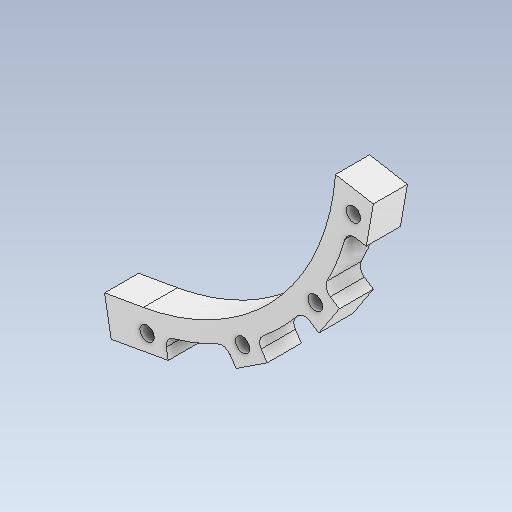
# Autodesk Inventor part: shell_5
Saved by Autodesk Inventor 2020 (Build 240168000, 168)
## iProperties
Created: 2020-07-15
Part Number: shell_5
Material: ABS Plastic
Document SubType Name: Modeling
Designer: psrobotics
Density: 1.06 g/cm^3
Appearance: Smooth - White
Author: psrobotics
Autodesk Inventor part; units mm, degrees
ref_plane "YZ Plane" through (0, 0, 0) normal (1, 0, 0) x (0, 1, 0)
ref_plane "XZ Plane" through (0, 0, 0) normal (0, 1, 0) x (-1, 0, 0)
ref_plane "XY Plane" through (0, 0, 0) normal (0, 0, 1) x (1, 0, 0)
sketch "Sketch1" plane through (0, 0, 0) normal (0, 0, 1) x (1, 0, 0)
  circle A0 centre (-48.56, 6.9152) radius 2.1 projected
  circle A1 centre (-32.9741, 22.501) radius 2.1 projected
  circle A2 centre (-69.0444, -1.2227) radius 2.1 projected
  circle A3 centre (-24.8362, 42.9855) radius 2.1 projected
  circle A4 centre (-46.3856, -8.3913) radius 8 projected
  line L0 (-28.6687, 48.4472) -> (-17.4995, 54.7179) projected
  arc A5 (-69.8258, 3.2089) -> (-28.6687, 48.4472) centre (-78.5082, 52.4493) ccw projected
  line L1 (-69.8258, 3.2089) -> (-78.128, 1.745) projected
  line L2 (-78.128, 1.745) -> (-74.0482, -21.3924) projected
  line L3 (-74.0482, -21.3924) -> (-70.3922, -20.7477) projected
  arc A6 (-70.3922, -20.7477) -> (-49.7861, -35.1763) centre (-46.3856, -8.3913) ccw projected
  line L4 (-49.7861, -35.1763) -> (-49.1414, -38.8323) projected
  line L5 (-49.1414, -38.8323) -> (-41.263, -37.4431) projected
  line L6 (-41.263, -37.4431) -> (4.3164, -53.3072) projected
  line L7 (4.3164, -53.3072) -> (1.8974, -59.9532) projected
  line L8 (1.8974, -59.9532) -> (17.5702, -63.2237) projected
  arc A7 (17.5702, -63.2237) -> (22.7521, -63.408) centre (22.2724, -3.9734) ccw projected
  line L9 (22.7521, -63.408) -> (22.7442, -62.4373) projected
  arc A8 (24.6597, -60.4229) -> (22.7442, -62.4373) centre (24.7442, -62.4211) ccw projected
  arc A9 (24.6597, -60.4229) -> (33.3265, -59.3815) centre (22.2724, -3.9734) ccw projected
  arc A10 (35.6646, -60.8847) -> (33.3265, -59.3815) centre (33.7178, -61.3428) ccw projected
  line L10 (35.6646, -60.8847) -> (35.9706, -62.1851) projected
  arc A11 (35.9706, -62.1851) -> (41.9803, -60.4344) centre (22.2724, -3.9734) ccw projected
  line L11 (41.9803, -60.4344) -> (52.856, -55.363) projected
  arc A12 (52.856, -55.363) -> (58.0602, -51.8846) centre (22.2724, -3.9734) ccw projected
  line L12 (58.0602, -51.8846) -> (57.2607, -50.8143) projected
  arc A13 (57.6121, -48.0569) -> (57.2607, -50.8143) centre (58.863, -49.6174) ccw projected
  arc A14 (57.6121, -48.0569) -> (63.9808, -42.0872) centre (22.2724, -3.9734) ccw projected
  arc A15 (66.7551, -41.9147) -> (63.9808, -42.0872) centre (65.4572, -43.4363) ccw projected
  line L13 (66.7551, -41.9147) -> (67.4937, -42.5447) projected
  arc A16 (67.4937, -42.5447) -> (70.6833, -38.4566) centre (22.2724, -3.9734) ccw projected
  line L14 (70.6833, -38.4566) -> (78.2523, -24.3484) projected
  line L15 (78.2523, -24.3484) -> (71.6063, -21.9294) projected
  arc A17 (71.6063, -21.9294) -> (67.7387, 22.2766) centre (22.2724, -3.9734) ccw projected
  line L16 (67.7387, 22.2766) -> (73.8637, 25.8129) projected
  line L17 (73.8637, 25.8129) -> (63.9599, 38.3925) projected
  arc A18 (63.9599, 38.3925) -> (60.1088, 41.8646) centre (22.2724, -3.9734) ccw projected
  line L18 (60.1088, 41.8646) -> (59.4908, 41.1159) projected
  arc A19 (56.7287, 40.804) -> (59.4908, 41.1159) centre (57.9484, 42.389) ccw projected
  arc A20 (56.7287, 40.804) -> (49.4201, 45.5771) centre (22.2724, -3.9734) ccw projected
  arc A21 (48.5953, 48.2316) -> (49.4201, 45.5771) centre (50.3811, 47.3311) ccw projected
  line L19 (48.5953, 48.2316) -> (49.1968, 49.4245) projected
  arc A22 (49.1968, 49.4245) -> (43.4677, 51.9463) centre (22.2724, -3.9734) ccw projected
  line L20 (43.4677, 51.9463) -> (31.8766, 55.0521) projected
  arc A23 (31.8766, 55.0521) -> (25.6541, 55.7327) centre (22.2724, -3.9734) ccw projected
  line L21 (25.6541, 55.7327) -> (25.5786, 54.3989) projected
  arc A24 (23.537, 52.5125) -> (25.5786, 54.3989) centre (23.5818, 54.512) ccw projected
  arc A25 (23.537, 52.5125) -> (14.821, 52.0331) centre (22.2724, -3.9734) ccw projected
  arc A26 (12.5849, 53.6843) -> (14.821, 52.0331) centre (14.5573, 54.0157) ccw projected
  line L22 (12.5849, 53.6843) -> (12.4241, 54.6417) projected
  arc A27 (12.4241, 54.6417) -> (7.3529, 53.5603) centre (22.2724, -3.9734) ccw projected
  line L23 (7.3529, 53.5603) -> (-7.5139, 47.618) projected
  line L24 (-7.5139, 47.618) -> (-17.4995, 54.7179) projected
  circle A28 centre (-71.296, -16.8454) radius 1.5 projected
  circle A29 centre (18.8152, -59.8032) radius 1.5 projected
  circle A30 centre (53.4562, -50.8504) radius 1.5 projected
  circle A31 centre (60.8075, 36.5725) radius 1.5 projected
  circle A32 centre (28.5162, 51.9811) radius 1.5 projected
  circle A33 centre (9.173, 50.4079) radius 1.5 projected
  circle A34 centre (44.8423, 47.6065) radius 1.5 projected
  circle A35 centre (67.2628, -37.2117) radius 1.5 projected
  circle A36 centre (38.1378, -57.9935) radius 1.5 projected
  circle A37 centre (-45.81, -34.6909) radius 1.5 projected
  circle A38 centre (22.2724, -3.9734) radius 32.5 projected
  circle A39 centre (-78.5082, 52.4493) radius 5.9 projected
  circle A40 centre (-78.5082, 52.4493) radius 50
  circle A41 centre (-78.5082, 52.4493) radius 54
  line L25 (-78.5082, 52.4493) -> (-69.0444, -1.2227)
  line L26 (-78.5082, 52.4493) -> (-24.8362, 42.9855)
  point P0 (0, 0)
  point P1 (-25.3286, 43.0723)
  point P2 (-29.2678, 43.7669)
  point P3 (-69.1312, -0.7303)
  dimension "d0" = 100
  dimension "d1" = 108
  constraints: 4 end point, 2 centre point, 2 coincident
  measures "d0" diameter of A40
  measures "d1" diameter of A41
extrude "Extrusion1" add sketch "Sketch1" along normal blind 7.3 contours A41 A0 | A0 A41 A2 L25 A5 L26 A3 A1 | A1 A41 | A41 L25 A2 | A3 L26 A41 picked at (-49.1962, 7.731) picked at (-33.8814, 22.9981) picked at (-68.8495, -0.1546) picked at (-25.9043, 42.7906)
sketch "Sketch2" plane through (0, 0, 7.3) normal (0, 0, 1) x (1, 0, 0)
  circle A0 centre (-48.56, 6.9152) radius 2.1 projected
  circle A1 centre (-32.9741, 22.501) radius 2.1 projected
  circle A2 centre (-69.0444, -1.2227) radius 2.1 projected
  circle A3 centre (-24.8362, 42.9855) radius 2.1 projected
  circle A4 centre (-46.3856, -8.3913) radius 8 projected
  line L0 (-28.6687, 48.4472) -> (-17.4995, 54.7179) projected
  arc A5 (-69.8258, 3.2089) -> (-28.6687, 48.4472) centre (-78.5082, 52.4493) ccw projected
  line L1 (-69.8258, 3.2089) -> (-78.128, 1.745) projected
  line L2 (-78.128, 1.745) -> (-74.0482, -21.3924) projected
  line L3 (-74.0482, -21.3924) -> (-70.3922, -20.7477) projected
  arc A6 (-70.3922, -20.7477) -> (-49.7861, -35.1763) centre (-46.3856, -8.3913) ccw projected
  line L4 (-49.7861, -35.1763) -> (-49.1414, -38.8323) projected
  line L5 (-49.1414, -38.8323) -> (-41.263, -37.4431) projected
  line L6 (-41.263, -37.4431) -> (4.3164, -53.3072) projected
  line L7 (4.3164, -53.3072) -> (1.8974, -59.9532) projected
  line L8 (1.8974, -59.9532) -> (17.5702, -63.2237) projected
  arc A7 (17.5702, -63.2237) -> (22.7521, -63.408) centre (22.2724, -3.9734) ccw projected
  line L9 (22.7521, -63.408) -> (22.7442, -62.4373) projected
  arc A8 (24.6597, -60.4229) -> (22.7442, -62.4373) centre (24.7442, -62.4211) ccw projected
  arc A9 (24.6597, -60.4229) -> (33.3265, -59.3815) centre (22.2724, -3.9734) ccw projected
  arc A10 (35.6646, -60.8847) -> (33.3265, -59.3815) centre (33.7178, -61.3428) ccw projected
  line L10 (35.6646, -60.8847) -> (35.9706, -62.1851) projected
  arc A11 (35.9706, -62.1851) -> (41.9803, -60.4344) centre (22.2724, -3.9734) ccw projected
  line L11 (41.9803, -60.4344) -> (52.856, -55.363) projected
  arc A12 (52.856, -55.363) -> (58.0602, -51.8846) centre (22.2724, -3.9734) ccw projected
  line L12 (58.0602, -51.8846) -> (57.2607, -50.8143) projected
  arc A13 (57.6121, -48.0569) -> (57.2607, -50.8143) centre (58.863, -49.6174) ccw projected
  arc A14 (57.6121, -48.0569) -> (63.9808, -42.0872) centre (22.2724, -3.9734) ccw projected
  arc A15 (66.7551, -41.9147) -> (63.9808, -42.0872) centre (65.4572, -43.4363) ccw projected
  line L13 (66.7551, -41.9147) -> (67.4937, -42.5447) projected
  arc A16 (67.4937, -42.5447) -> (70.6833, -38.4566) centre (22.2724, -3.9734) ccw projected
  line L14 (70.6833, -38.4566) -> (78.2523, -24.3484) projected
  line L15 (78.2523, -24.3484) -> (71.6063, -21.9294) projected
  arc A17 (71.6063, -21.9294) -> (67.7387, 22.2766) centre (22.2724, -3.9734) ccw projected
  line L16 (67.7387, 22.2766) -> (73.8637, 25.8129) projected
  line L17 (73.8637, 25.8129) -> (63.9599, 38.3925) projected
  arc A18 (63.9599, 38.3925) -> (60.1088, 41.8646) centre (22.2724, -3.9734) ccw projected
  line L18 (60.1088, 41.8646) -> (59.4908, 41.1159) projected
  arc A19 (56.7287, 40.804) -> (59.4908, 41.1159) centre (57.9484, 42.389) ccw projected
  arc A20 (56.7287, 40.804) -> (49.4201, 45.5771) centre (22.2724, -3.9734) ccw projected
  arc A21 (48.5953, 48.2316) -> (49.4201, 45.5771) centre (50.3811, 47.3311) ccw projected
  line L19 (48.5953, 48.2316) -> (49.1968, 49.4245) projected
  arc A22 (49.1968, 49.4245) -> (43.4677, 51.9463) centre (22.2724, -3.9734) ccw projected
  line L20 (43.4677, 51.9463) -> (31.8766, 55.0521) projected
  arc A23 (31.8766, 55.0521) -> (25.6541, 55.7327) centre (22.2724, -3.9734) ccw projected
  line L21 (25.6541, 55.7327) -> (25.5786, 54.3989) projected
  arc A24 (23.537, 52.5125) -> (25.5786, 54.3989) centre (23.5818, 54.512) ccw projected
  arc A25 (23.537, 52.5125) -> (14.821, 52.0331) centre (22.2724, -3.9734) ccw projected
  arc A26 (12.5849, 53.6843) -> (14.821, 52.0331) centre (14.5573, 54.0157) ccw projected
  line L22 (12.5849, 53.6843) -> (12.4241, 54.6417) projected
  arc A27 (12.4241, 54.6417) -> (7.3529, 53.5603) centre (22.2724, -3.9734) ccw projected
  line L23 (7.3529, 53.5603) -> (-7.5139, 47.618) projected
  line L24 (-7.5139, 47.618) -> (-17.4995, 54.7179) projected
  circle A28 centre (-71.296, -16.8454) radius 1.5 projected
  circle A29 centre (18.8152, -59.8032) radius 1.5 projected
  circle A30 centre (53.4562, -50.8504) radius 1.5 projected
  circle A31 centre (60.8075, 36.5725) radius 1.5 projected
  circle A32 centre (28.5162, 51.9811) radius 1.5 projected
  circle A33 centre (9.173, 50.4079) radius 1.5 projected
  circle A34 centre (44.8423, 47.6065) radius 1.5 projected
  circle A35 centre (67.2628, -37.2117) radius 1.5 projected
  circle A36 centre (38.1378, -57.9935) radius 1.5 projected
  circle A37 centre (-45.81, -34.6909) radius 1.5 projected
  circle A38 centre (22.2724, -3.9734) radius 32.5 projected
  line L25 (-78.5082, 52.4493) -> (-69.0444, -1.2227)
  line L26 (-64.4974, -3.975) -> (-72.3759, -5.3642)
  line L27 (-72.3759, -5.3642) -> (-73.5914, 1.5295)
  line L28 (-73.5914, 1.5295) -> (-65.7129, 2.9187)
  line L29 (-65.7129, 2.9187) -> (-64.4974, -3.975)
  line L30 (-64.4974, -3.975) -> (-73.5914, 1.5295) construction
  line L31 (-72.3759, -5.3642) -> (-65.7129, 2.9187) construction
  line L32 (-43.2948, 6.189) -> (-49.9787, 1.793)
  line L33 (-47.1413, 12.0374) -> (-43.2948, 6.189)
  line L34 (-53.8252, 7.6414) -> (-47.1413, 12.0374)
  line L35 (-49.9787, 1.793) -> (-53.8252, 7.6414)
  line L36 (-27.8519, 23.9197) -> (-32.248, 17.2358)
  line L37 (-33.7003, 27.7663) -> (-27.8519, 23.9197)
  line L38 (-38.0964, 21.0824) -> (-33.7003, 27.7663)
  line L39 (-32.248, 17.2358) -> (-38.0964, 21.0824)
  line L40 (-20.6948, 46.3169) -> (-22.084, 38.4385)
  line L41 (-27.5884, 47.5325) -> (-20.6948, 46.3169)
  line L42 (-28.9776, 39.654) -> (-27.5884, 47.5325)
  line L43 (-22.084, 38.4385) -> (-28.9776, 39.654)
  line L44 (-72.3759, -5.3642) -> (-76.7388, -6.1335)
  line L45 (-28.6687, 48.4472) -> (-20.5709, 47.0193)
  line L46 (-20.5709, 47.0193) -> (-20.6948, 46.3169)
  line L47 (-25.3286, 43.0723) -> (-29.2678, 43.7669) projected
  point P0 (0, 0)
  point P1 (-69.6522, 2.2241)
  point P2 (-28.283, 43.5932)
  dimension "d4" = 8
  dimension "d5" = 7
  dimension "d8" = 70
  constraints: 44 end point, 4 perpendicular, 3 parallel, 2 midpoint, 1 point on line, 25 other
  measures "d4" distance of L26.start L26.end
  measures "d5" distance of L26.end L27.end
extrude "Extrusion2" add sketch "Sketch2" against normal blind 7.3 contours A0 | A1 | A2 | L28 L29 L26 L27 | L28 L27 L44 L2 L1 L25 | A5 L45 L46 L41 L42 L47 | L42 L41 L40 L43 | A3 | L32 L35 L34 L33 | L36 L39 L38 L37
sketch "Sketch3" plane through (0, 0, 7.3) normal (0, 0, 1) x (1, 0, 0)
  circle A0 centre (-24.8362, 42.9855) radius 2.1 projected
  circle A1 centre (-32.9741, 22.501) radius 2.1 projected
  circle A2 centre (-48.56, 6.9152) radius 2.1 projected
  circle A3 centre (-69.0444, -1.2227) radius 2.1 projected
  point P0 (0, 0)
hole "Hole1" at (-24.8362, 42.9855, 7.3) at (-32.9741, 22.501, 7.3) at (-48.56, 6.9152, 7.3) at (-69.0444, -1.2227, 7.3) direction (0, 0, -1) diameter 3.1 depth 17
fillet "Fillet1" radius 2 6 edges at (-65.2178, 0.1104, 3.65) (-52.2582, 5.2588, 3.65) (-45.5743, 9.6549, 3.65) (-35.7139, 19.5154, 3.65) (-31.3178, 26.1993, 3.65) (-26.1693, 39.1588, 3.65)
body "Solid1"
